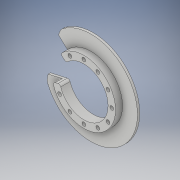
# Autodesk Inventor part: RotateLimitPlate
Saved by Autodesk Inventor 2018.3 (Build 223284000, 284)
## iProperties
Created: 2019-09-02
Part Number: RotateLimitPlate
Material: Generic
Document SubType Name: Modeling
Designer: Srinity
Density: 1 g/cm^3
Appearance: Default
Author: Srinity
Autodesk Inventor part; units mm, degrees
ref_plane "YZ Plane" through (0, 0, 0) normal (1, 0, 0) x (0, 1, 0)
ref_plane "XZ Plane" through (0, 0, 0) normal (0, 1, 0) x (-1, 0, 0)
ref_plane "XY Plane" through (0, 0, 0) normal (0, 0, 1) x (1, 0, 0)
sketch "Sketch1" plane through (0, 0, 0) normal (0, 0, 1) x (1, 0, 0)
  circle A0 centre (0, 38.1) radius 2.54
  circle A1 centre (-19.05, 32.9956) radius 2.54
  circle A2 centre (-32.9956, 19.05) radius 2.54
  circle A3 centre (-38.1, 0) radius 2.54
  arc A4 (-34.7393, -15.6458) -> (-25.6134, 28.2057) centre (0, 0) ccw
  line L0 (0, 0) -> (-22.4665, 0)
  arc A5 (-42.1565, -9.3459) -> (-31.8356, 29.172) centre (0, 0) ccw
  arc A6 (-32.2373, -7.1468) -> (-24.3449, 22.308) centre (0, 0) ccw
  line L1 (-31.8356, 29.172) -> (-24.3449, 22.308)
  line L2 (-42.1565, -9.3459) -> (-32.2373, -7.1468)
  circle A7 centre (-32.9956, -19.05) radius 2.54
  circle A8 centre (-19.05, -32.9956) radius 2.54
  circle A9 centre (0, -38.1) radius 2.54
  circle A10 centre (19.05, -32.9956) radius 2.54
  circle A11 centre (32.9956, -19.05) radius 2.54
  circle A12 centre (38.1, 0) radius 2.54
  circle A13 centre (32.9956, 19.05) radius 2.54
  circle A14 centre (19.05, 32.9956) radius 2.54
  dimension "d0" = 38.1
  dimension "d3" = 360
  dimension "d5" = 5.08
  dimension "d6" = 5.08
  dimension "d7" = 5.08
  dimension "d8" = 55
  dimension "d9" = 42.5
  constraints: 15 centre point, 7 point on circle, 6 end point, 2 point on line, 1 coincident, 1 horizontal, 1 vertical alignment, 25 other
  measures "d0" distance of point (0, 0) A0.centre
  measures "d5" diameter of A0
  measures "d6" radial gap between concentric circles of A4 A5
  measures "d7" radial gap between concentric circles of A6 A4
  measures "d8" angle of L2 L1
  measures "d9" angle of L1 L0
extrude "Extrusion1" add sketch "Sketch1" along normal blind 12.7 contours L2 A6 L1 A5
fillet "Fillet2" radius 3.175 4 edges at (-31.8356, 29.172, 6.35) (-24.3449, 22.308, 6.35) (-32.2373, -7.1468, 6.35) (-42.1565, -9.3459, 6.35)
sketch "Sketch2" plane through (0, 0, 0) normal (0, 0, -1) x (-1, 0, 0)
  arc A0 (29.42, 31.6066) -> (41.2817, -12.6621) centre (0, 0) ccw projected
  arc A1 (46.8171, 42.9) -> (61.9948, -13.7439) centre (0, 0) ccw
  line L0 (46.8171, 42.9) -> (29.4017, 26.9417)
  line L1 (29.4017, 26.9417) -> (26.5829, 24.3587) projected
  arc A2 (29.4017, 26.9417) -> (29.42, 31.6066) centre (27.2567, 29.2826) ccw projected
  line L2 (35.2008, -7.8038) -> (38.9335, -8.6314) projected
  arc A3 (41.2817, -12.6621) -> (38.9335, -8.6314) centre (38.2463, -11.7311) ccw projected
  line L3 (61.9948, -13.7439) -> (38.9335, -8.6314)
  dimension "d20" = 63.5
  constraints: 4 end point, 2 collinear, 2 point on circle, 1 centre point
  measures "d20" radius of A1
extrude "Extrusion2" add sketch "Sketch2" against normal blind 3.175
chamfer "Chamfer3" distance 7.62 distance2 3.81 1 edges at (-46.8171, 42.9, 1.5875) measured on face at (-46.4779, 43.2673, 1.5875)
chamfer "Chamfer4" distance 3.81 distance2 7.62 1 edges at (-61.9948, -13.7439, 1.5875) measured on face at (-61.5066, -13.6357, 1.5875)
fillet "Fillet3" radius 12.7 2 edges at (-59.9021, -21.0709, 1.5875) (-41.3413, 48.199, 1.5875)
equation "\"d7\" = d6"
body "Solid1"
